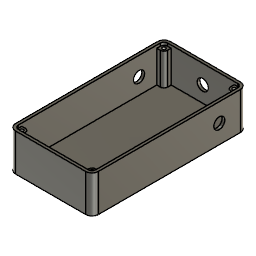
bottom_shield (Autodesk Fusion 360 design; units mm, degrees)
part number: 2025-12-11-09-13-35-348
Autodesk Fusion 360 part; units mm, degrees
sketch "Esquisse1" plane through (0, 0, 0) normal (0, 0, 1) x (1, 0, 0)
  line L0 (4.6, 0) -> (55.4, 0)
  line L1 (60, -4.6) -> (60, -107.4)
  line L2 (55.4, -112) -> (4.6, -112)
  line L3 (0, -107.4) -> (0, -4.6)
  arc A0 (1, 0) -> (0, -1) centre (1, -1) ccw
  arc A1 (60, -1) -> (59, 0) centre (59, -1) ccw
  arc A2 (59, -112) -> (60, -111) centre (59, -111) ccw
  arc A3 (0, -111) -> (1, -112) centre (1, -111) ccw
  arc A4 (4.6, 0) -> (0, -4.6) centre (4.6, -4.6) ccw
  arc A5 (55.4, -112) -> (60, -107.4) centre (55.4, -107.4) ccw
  arc A6 (60, -4.6) -> (55.4, 0) centre (55.4, -4.6) ccw
  arc A7 (0, -107.4) -> (4.6, -112) centre (4.6, -107.4) ccw
  point P0 (60, 0)
  point P1 (0, -112)
  dimension "d1" = 60
  dimension "d2" = 112
  dimension "d3" = 1
  dimension "d4" = 4.6
  constraint horizontal L0
  constraint vertical L1
  constraint horizontal L2
  constraint vertical L3
  constraint coincident origin L0
  constraint coincident origin L3
  constraint tangent L0 A0
  constraint tangent L3 A0
  constraint coincident P0 L0
  constraint coincident P0 L1
  constraint tangent L0 A1
  constraint tangent L1 A1
  constraint equal A0 A1
  constraint tangent L1 A2
  constraint tangent L2 A2
  constraint equal A0 A2
  constraint coincident P1 L3
  constraint coincident P1 L2
  constraint tangent L3 A3
  constraint tangent L2 A3
  constraint equal A0 A3
  constraint coincident L0 A0.start
  constraint coincident L3 A0.end
  constraint tangent L0 A4
  constraint tangent L3 A4
  constraint coincident L2 A2.start
  constraint coincident L1 A2.end
  constraint tangent L2 A5
  constraint tangent L1 A5
  constraint equal A4 A5
  constraint coincident L0 A1.end
  constraint coincident L1 A1.start
  constraint tangent L0 A6
  constraint tangent L1 A6
  constraint equal A4 A6
  constraint coincident L3 A3.start
  constraint coincident L2 A3.end
  constraint tangent L3 A7
  constraint tangent L2 A7
  constraint equal A4 A7
  measures "d1" distance of origin P0
  measures "d2" distance of origin P1
  measures "d3" radius of A0
  measures "d4" radius of A4
extrude "Extrusion1" add sketch "Esquisse1" along normal blind 2
shell "Coque1" thickness 25 removed faces 1 at (40, -38.8667, 2)
sketch "Esquisse2" plane through (0, 0, 2) normal (0, 0, 1) x (-1, 0, 0)
  arc A0 (-4.6, 0) -> (0, 4.6) centre (-4.6, 4.6) ccw
  line L0 (0, 4.6) -> (0, 107.4)
  arc A1 (0, 107.4) -> (-4.6, 112) centre (-4.6, 107.4) ccw
  line L1 (-4.6, 112) -> (-55.4, 112)
  arc A2 (-55.4, 112) -> (-60, 107.4) centre (-55.4, 107.4) ccw
  line L2 (-60, 107.4) -> (-60, 4.6)
  arc A3 (-60, 4.6) -> (-55.4, 0) centre (-55.4, 4.6) ccw
  line L3 (-55.4, 0) -> (-4.6, 0)
  line L4 (-4.6, 110) -> (-55.4, 110)
  arc A4 (-55.4, 110) -> (-58, 107.4) centre (-55.4, 107.4) ccw
  line L5 (-58, 107.4) -> (-58, 4.6)
  arc A5 (-58, 4.6) -> (-55.4, 2) centre (-55.4, 4.6) ccw
  line L6 (-55.4, 2) -> (-4.6, 2)
  arc A6 (-4.6, 2) -> (-2, 4.6) centre (-4.6, 4.6) ccw
  line L7 (-2, 4.6) -> (-2, 107.4)
  arc A7 (-2, 107.4) -> (-4.6, 110) centre (-4.6, 107.4) ccw
  dimension "d8" = -2
extrude "Extrusion2" add sketch "Esquisse2" along normal blind 25
sketch "Esquisse3" plane through (0, 0, 2) normal (0, 0, 1) x (-1, 0, 0)
  line L0 (-4.6, 110) -> (-55.4, 110)
  arc A0 (-55.4, 110) -> (-58, 107.4) centre (-55.4, 107.4) ccw
  line L1 (-58, 107.4) -> (-58, 4.6)
  arc A1 (-58, 4.6) -> (-55.4, 2) centre (-55.4, 4.6) ccw
  line L2 (-55.4, 2) -> (-4.6, 2)
  arc A2 (-4.6, 2) -> (-2, 4.6) centre (-4.6, 4.6) ccw
  line L3 (-2, 4.6) -> (-2, 107.4)
  arc A3 (-2, 107.4) -> (-4.6, 110) centre (-4.6, 107.4) ccw
  line L4 (-7.2, 2) -> (-7.2, 4.6)
  line L5 (-4.6, 7.2) -> (-2, 7.2)
  arc A4 (-4.6, 2) -> (-2, 4.6) centre (-4.6, 4.6) ccw
  arc A5 (-4.6, 7.2) -> (-7.2, 4.6) centre (-4.6, 4.6) ccw
  line L6 (-2, 104.8) -> (-4.6, 104.8)
  line L7 (-7.2, 107.4) -> (-7.2, 110)
  arc A6 (-7.2, 107.4) -> (-4.6, 104.8) centre (-4.6, 107.4) ccw
  arc A7 (-2, 107.4) -> (-4.6, 110) centre (-4.6, 107.4) ccw
  line L8 (-58, 104.8) -> (-55.4, 104.8)
  line L9 (-52.8, 107.4) -> (-52.8, 110)
  arc A8 (-55.4, 110) -> (-58, 107.4) centre (-55.4, 107.4) ccw
  arc A9 (-55.4, 104.8) -> (-52.8, 107.4) centre (-55.4, 107.4) ccw
  line L10 (-52.8, 2) -> (-52.8, 4.6)
  line L11 (-55.4, 7.2) -> (-58, 7.2)
  arc A10 (-52.8, 4.6) -> (-55.4, 7.2) centre (-55.4, 4.6) ccw
  arc A11 (-58, 4.6) -> (-55.4, 2) centre (-55.4, 4.6) ccw
  dimension "d11" = 2.6
  dimension "d12" = 2.6
  dimension "d13" = 5.2
  constraint coincident L2 L4.start
  constraint perpendicular L2 L4
  constraint coincident L3 L5.end
  constraint perpendicular L3 L5
  constraint tangent L4 A4
  constraint tangent L5 A4
  constraint coincident L5.start A4
  constraint concentric A4 A5
  constraint concentric A1 A10
  constraint concentric A0 A8
  constraint concentric A3 A6
  constraint coincident L3 L6.start
  constraint perpendicular L3 L6
  constraint coincident L0 L7.end
  constraint perpendicular L0 L7
  constraint tangent L6 A6
  constraint tangent L7 A6
  constraint concentric A6 A7
  constraint coincident L1 L8.start
  constraint perpendicular L1 L8
  constraint coincident L0 L9.end
  constraint perpendicular L0 L9
  constraint tangent L8 A8
  constraint tangent L9 A8
  constraint coincident L8.end A8
  constraint concentric A8 A9
  constraint coincident L2 L10.start
  constraint perpendicular L2 L10
  constraint coincident L1 L11.end
  constraint perpendicular L1 L11
  constraint tangent L10 A10
  constraint tangent L11 A10
  constraint concentric A10 A11
  measures "d11" distance of L2 A2.centre
  measures "d12" distance of L3 A2.centre
  measures "d13" diameter of A4
extrude "Extrusion3" add sketch "Esquisse3" along normal blind 23 contours L0 L3 A3 L6 L7 A6 A7 | L0 A0 L1 L8 L9 A8 A9 | L2 A2 L3 L4 L5 A4 A5 | L1 A1 L2 L10 L11 A10 A11
sketch "Esquisse4" plane through (0, 0, 25) normal (0, 0, 1) x (-1, 0, 0)
  arc A0 (-58, 4.6) -> (-55.4, 2) centre (-55.4, 4.6) ccw
  line L0 (-55.4, 2) -> (-52.8, 2)
  line L1 (-52.8, 2) -> (-52.8, 4.6)
  arc A1 (-52.8, 4.6) -> (-55.4, 7.2) centre (-55.4, 4.6) ccw
  line L2 (-55.4, 7.2) -> (-58, 7.2)
  line L3 (-58, 7.2) -> (-58, 4.6)
hole "Perçage1" at (55.4, -4.6, 25) direction (0, 0, -1) diameter 2.529 depth 10 tip angle 118
thread "Filetage1" "ISO Metric profile 3.0 M3x0.5 M3x0.5 6H" thread offset 0 thread depth 7.4
sketch "Esquisse5" plane through (0, 0, 25) normal (0, 0, 1) x (-1, 0, 0)
  line L0 (-7.2, 2) -> (-4.6, 2)
  arc A0 (-4.6, 2) -> (-2, 4.6) centre (-4.6, 4.6) ccw
  line L1 (-2, 4.6) -> (-2, 7.2)
  line L2 (-2, 7.2) -> (-4.6, 7.2)
  arc A1 (-4.6, 7.2) -> (-7.2, 4.6) centre (-4.6, 4.6) ccw
  line L3 (-7.2, 4.6) -> (-7.2, 2)
hole "Perçage2" at (4.6, -4.6, 25) direction (0, 0, -1) diameter 2.529 depth 10 tip angle 118
thread "Filetage2" "ISO Metric profile 3.0 M3x0.5 M3x0.5 6H" thread offset 0 thread depth 7.4
sketch "Esquisse6" plane through (0, 0, 25) normal (0, 0, 1) x (-1, 0, 0)
  line L0 (-2, 104.8) -> (-2, 107.4)
  arc A0 (-2, 107.4) -> (-4.6, 110) centre (-4.6, 107.4) ccw
  line L1 (-4.6, 110) -> (-7.2, 110)
  line L2 (-7.2, 110) -> (-7.2, 107.4)
  arc A1 (-7.2, 107.4) -> (-4.6, 104.8) centre (-4.6, 107.4) ccw
  line L3 (-4.6, 104.8) -> (-2, 104.8)
hole "Perçage3" at (4.6, -107.4, 25) direction (0, 0, -1) diameter 2.529 depth 10 tip angle 118
thread "Filetage3" "ISO Metric profile 3.0 M3x0.5 M3x0.5 6H" thread offset 0 thread depth 7.4
sketch "Esquisse7" plane through (0, 0, 25) normal (0, 0, 1) x (-1, 0, 0)
  arc A0 (-55.4, 104.8) -> (-52.8, 107.4) centre (-55.4, 107.4) ccw
  line L0 (-52.8, 107.4) -> (-52.8, 110)
  line L1 (-52.8, 110) -> (-55.4, 110)
  arc A1 (-55.4, 110) -> (-58, 107.4) centre (-55.4, 107.4) ccw
  line L2 (-58, 107.4) -> (-58, 104.8)
  line L3 (-58, 104.8) -> (-55.4, 104.8)
hole "Perçage4" at (55.4, -107.4, 25) direction (0, 0, -1) diameter 2.529 depth 10 tip angle 118
thread "Filetage4" "ISO Metric profile 3.0 M3x0.5 M3x0.5 6H" thread offset 0 thread depth 7.4
sketch "Esquisse10" plane through (0, 0, 0) normal (-1, 0, 0) x (0, -1, 0)
  line L0 (4.6, 0) -> (107.4, 0)
  line L1 (107.4, 0) -> (107.4, 27)
  line L2 (107.4, 27) -> (4.6, 27)
  line L3 (4.6, 27) -> (4.6, 0)
  circle A0 centre (20, 13.5) radius 4
  point P0 (0, 27)
  dimension "d58" = 8
  dimension "d59" = 13.5
  dimension "d60" = 20
  measures "d58" diameter of A0
  measures "d59" distance of L2 A0.centre
  measures "d60" horizontal distance of A0.centre P0
extrude "Extrusion4" cut sketch "Esquisse10" against normal blind 68 contours A0
sketch "Esquisse11" plane through (0, 0, 0) normal (0, 1, 0) x (-1, 0, 0)
  line L0 (-55.4, 0) -> (-4.6, 0)
  line L1 (-4.6, 0) -> (-4.6, 27)
  line L2 (-4.6, 27) -> (-55.4, 27)
  line L3 (-55.4, 27) -> (-55.4, 0)
  circle A0 centre (-30, 13.5) radius 4
  dimension "d63" = 8
  dimension "d64" = 25.4
  dimension "d65" = 13.5
  measures "d63" diameter of A0
  measures "d64" distance of L1 A0.centre
  measures "d65" distance of L2 A0.centre
extrude "Extrusion5" cut sketch "Esquisse11" against normal blind 24 contours A0
equation "d65 = ( 27 / 2 ) * 1 mm"
